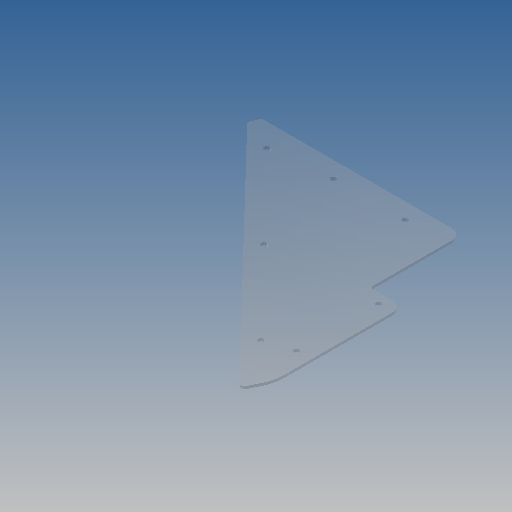
# Autodesk Inventor part: J009838
Saved by Autodesk Inventor 2020.3 (Build 243373000, 373)
## iProperties
RuleStatus: InUse
AfterDocSave0: file://Part Number Cleaner
Created: 2019-12-20
Material: Polycarbonate, Clear
Vendor: HHMI: JRC - ID&F
Document SubType Name: Sheet Metal
Designer: goulett
Density: 1.2 g/cm^3
Appearance: Polycarbonate - Clear
Part Number: J009838
Project: P-342901
Description: LEFT SIDE RAT CAGE PANEL REPAIR
Sheet Metal Rule: Default
LAB/DEPT: VIVARIUM (SHARED RESOURCES)
REQUESTING SCIENTIST: COX, JAMES
SURFACE ROUGHNESS: N/A
DESIGN DEPARTMENT: HHMI: JRC - ID&F
SPECIAL FINISH: N/A
ALTERED ITEM PART NUMBER: N/A
ALTERED ITEM VENDOR: N/A
ALTERED ITEM DESCRIPTION: N/A
Author: goulett
Revision Number: -
Autodesk Inventor part; units mm, degrees
ref_plane "YZ Plane" through (0, 0, 0) normal (1, 0, 0) x (0, 1, 0)
ref_plane "XZ Plane" through (0, 0, 0) normal (0, 1, 0) x (-1, 0, 0)
ref_plane "XY Plane" through (0, 0, 0) normal (0, 0, 1) x (1, 0, 0)
sketch "Sketch1" plane through (0, 0, 0) normal (0, 1, 0) x (-1, 0, 0)
  line L0 (0, 0) -> (-20.32, 0)
  line L1 (-20.32, 0) -> (-20.32, 79.6462)
  line L2 (-20.32, 79.6462) -> (-13.0825, 94.4853)
  line L3 (133.35, -57.15) -> (0, -57.15)
  line L4 (0, -57.15) -> (0, 0)
  line L5 (25.4, -46.99) -> (69.85, -46.99) construction
  line L6 (107.0012, -42.6627) -> (5.5464, 62.3969) construction
  line L7 (-11.43, 57.15) -> (-11.43, 6.35) construction
  line L8 (164.084, 0) -> (-51.054, 0) construction
  line L9 (133.35, -57.15) -> (-13.0825, 94.4853)
  line L10 (107.0012, -42.6627) -> (113.3962, -36.4872) construction
  point P0 (56.2738, 9.8671)
  dimension "d25" = 50.8
  dimension "d26" = 146.05
  dimension "d27" = 73.025
  dimension "d28" = 44.45
  dimension "d32" = 57.15
  dimension "d33" = 133.35
  dimension "d44" = 20.32
  dimension "d46" = 8.89
  dimension "d47" = 10.16
  dimension "d49" = 25.4
  dimension "d60" = 46
  dimension "d61" = 8.89
  dimension "d64" = 6.35
  dimension "d66" = 28.7247
  dimension "d71" = 70
  dimension "d72" = 16.51
  constraints: 20 end point, 4 perpendicular, 2 vertical, 1 horizontal, 1 midpoint, 1 parallel, 1 point on line
  measures "d25" distance of L7.start L7.end
  measures "d26" distance of L6.start L6.end
  measures "d27" distance of point (56.274, 9.867) L6.end
  measures "d28" distance of L5.start L5.end
  measures "d32" distance of L0.start L3.end
  measures "d33" distance of L3.start L3.end
  measures "d44" distance between parallel lines of L1 L4
  measures "d46" distance between parallel lines of L9 L6
  measures "d47" distance between parallel lines of L3 L5
  measures "d49" distance from line of L4 L5.start
  measures "d60" angle of L9 L3
  measures "d61" distance between parallel lines of L1 L7
  measures "d64" distance from line of L0 L7.end
  measures "d66" distance from line of L3.start L10
  measures "d71" angle of L9 L2
  measures "d72" distance of L1.end L2.end
extrude "Plate1" add sketch "Sketch1" along normal blind 1.5875
hole "Hole1" at (-5.5464, 0, 62.3969) at (11.43, 0, 57.15) at (-56.2738, 0, 9.8671) at (-107.0012, 0, -42.6627) at (-69.85, 0, -46.99) at (-25.4, 0, -46.99) at (11.43, 0, 6.35) direction (0, 1, 0) diameter 3.4544 end through all
chamfer "Corner Chamfer1" distance 8.89 angle 45 1 edges at (-133.35, 0.7937, -57.15)
fillet "Corner Round1" radius 6.35 2 edges at (20.32, 0.7937, 0) (0, 0.7937, -57.15)
fillet "Corner Round1" radius 2.54 3 edges at (13.0825, 0.7937, 94.4853) (-127.1745, 0.7937, -50.7551) (-124.46, 0.7937, -57.15)
fillet "Corner Round1" radius 1.27 1 edges at (0, 0.7937, 0)
fillet "Corner Round1" radius 25.4 1 edges at (20.32, 0.7937, 79.6462)
equation "\"d27\" = 0.5 * d26"
equation "\"BendReliefWidth\" = Thickness"
equation "\"BendReliefDepth\" = 0.5 * Thickness"
equation "\"MinimumRemnant\" = 2 * Thickness"
equation "\"GapSize\" = Thickness"
equation "\"Thickness\" = 1.5875"
body "Solid2"
